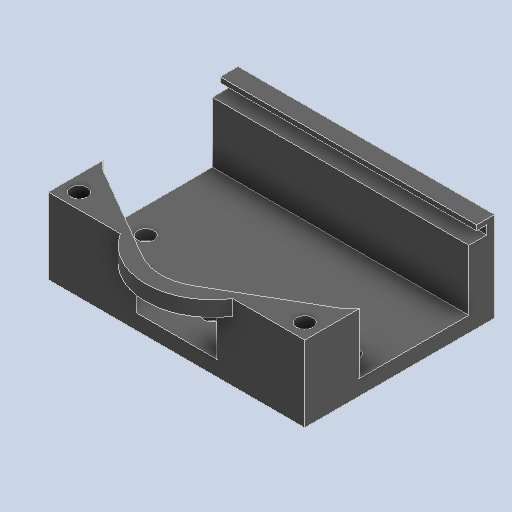
# Autodesk Inventor part: belt_cover_middle
Saved by Autodesk Inventor 2024.1 (Build 281209000, 209)
## iProperties
Created: 2025-02-03
Part Number: belt_cover_middle
Material: 一般
Document SubType Name: モデリング
Designer: hibik
Density: 1 g/cm^3
Appearance: 既定
Sheet Metal Rule: Default_mm
Author: hibik
Autodesk Inventor part; units mm, degrees
ref_plane "YZ Plane" through (0, 0, 0) normal (1, 0, 0) x (0, 1, 0)
ref_plane "XZ Plane" through (0, 0, 0) normal (0, 1, 0) x (-1, 0, 0)
ref_plane "XY Plane" through (0, 0, 0) normal (0, 0, 1) x (1, 0, 0)
sketch "スケッチ1" plane through (0, 0, 0) normal (0, 1, 0) x (-1, 0, 0)
  line L0 (75, 0) -> (105, -51.9615)
  line L1 (-75, 0) -> (-105, -51.9615)
  line L2 (0, -218.2384) -> (0, 36.3731)
  line L3 (147, 0) -> (-147, 0)
  line L4 (105, -51.9615) -> (30, -181.8653)
  line L5 (30, -181.8653) -> (-30, -181.8653)
  line L6 (-30, -181.8653) -> (-105, -51.9615)
  line L7 (75, 0) -> (-75, 0)
  line L8 (34, 0) -> (34, -24.3509)
  line L9 (34, -24.3509) -> (48.7058, -49.822)
  line L10 (48.7058, -49.822) -> (90, -25.9808)
  line L11 (45, 0) -> (45, -18) construction
  line L12 (45, -18) -> (34, -24.3509) construction
  line L13 (84.5, -87.4686) -> (63.4115, -75.2931)
  line L14 (63.4115, -75.2931) -> (48.7058, -49.822)
  line L15 (-34, 0) -> (-34, -24.3509)
  line L16 (-34, -24.3509) -> (-48.7058, -49.822)
  line L17 (-63.4115, -75.2931) -> (-48.7058, -49.822)
  line L18 (-84.5, -87.4686) -> (-63.4115, -75.2931)
  circle A0 centre (30, -32.75) radius 1.6
  circle A1 centre (-30, -32.75) radius 1.6
  line L19 (35.5295, -27) -> (-35.5295, -27)
  point P0 (0, 0)
  point P1 (0, 0)
  point P2 (0, -27)
  dimension "d1" = 150
  dimension "d2" = 60
  dimension "d3" = 60
  dimension "d6" = 60
  dimension "d30" = 60
  dimension "d31" = 18
  dimension "d32" = 30
  dimension "d33" = 41
  dimension "d34" = 3.2
  dimension "d35" = 30
  dimension "d36" = 32.75
  dimension "d37" = 27
  measures "d1" distance of L1.start L0.start
  measures "d2" angle of L3 L0
  measures "d3" angle of L1 L3
  measures "d6" distance of L4.end L5.end
  measures "d30" angle of L11 L12
  measures "d31" distance of L11.start L11.end
  measures "d32" distance of L0.start L11.start
  measures "d33" distance of L0.start L8.start
  measures "d34" diameter of A0
  measures "d35" distance from line of L2 A0.centre
  measures "d36" distance from line of L7 A0.centre
  measures "d37" distance between parallel lines of L7 L19
extrude "プレート1" add sketch "スケッチ1" along normal blind 1.5 contours L14 L13 L4 L5 L2 L19 L9 | L2 L5 L6 L18 L17 L16 L19
sketch "スケッチ4" plane through (0, 1.5, 0) normal (0, 1, 0) x (1, 0, 0)
  circle A0 centre (30, 67.8013) radius 1.6 projected
  circle A1 centre (45, 67.8013) radius 1.6 projected
  line L0 (0, 218.2384) -> (0, -36.3731) projected
  circle A2 centre (-30, 67.8013) radius 1.6
  circle A3 centre (-45, 67.8013) radius 1.6
  line L1 (61.6173, 73.1025) -> (25, 73.1025) projected
  line L2 (25, 73.1025) -> (25, 62.5) projected
  line L3 (-61.6173, 73.1025) -> (-25, 73.1025) projected
  line L4 (-25, 73.1025) -> (-25, 62.5) projected
  line L5 (-25, 62.5) -> (25, 62.5)
  line L6 (-30, 73.1025) -> (30, 73.1025)
  line L7 (30, 73.1025) -> (30, 181.8653)
  line L8 (30, 181.8653) -> (-30, 181.8653)
  line L9 (-30, 181.8653) -> (-30, 73.1025)
  line L10 (-25, 62.5) -> (25, 62.5)
  line L11 (25, 62.5) -> (25, 73.1025)
  line L12 (25, 73.1025) -> (-25, 73.1025)
  line L13 (-25, 73.1025) -> (-25, 62.5)
  line L14 (30, 181.8653) -> (84.5, 87.4686) projected
  line L15 (70, 112.5833) -> (30, 89.4893)
  line L16 (-30, 89.4893) -> (-70, 112.5833)
  line L17 (-84.5, 87.4686) -> (-30, 181.8653) projected
  line L18 (84.5, 87.4686) -> (63.4115, 75.2931) projected
  line L19 (-63.4115, 75.2931) -> (-84.5, 87.4686) projected
  line L20 (-35.5295, 27) -> (-63.4115, 75.2931) projected
  point P0 (0, 0)
  dimension "d40" = 80
  constraints: 22 end point, 6 parallel, 5 point on line, 3 horizontal, 2 centre point, 2 equal radius, 2 perpendicular, 2 symmetric about line, 1 coincident, 1 horizontal alignment
  measures "d40" distance from line of L14.start L15
extrude "切り取り3" cut sketch "スケッチ4" against normal blind 1.5
sketch "スケッチ5" plane through (0, 1.5, 0) normal (0, 1, 0) x (1, 0, 0)
  line L0 (-75, 44) -> (75, 44) projected
  circle A0 centre (-20, 41) radius 3
  circle A1 centre (20, 41) radius 3
  line L1 (-25, 62.5) -> (25, 62.5) projected
  line L2 (0, 62.5) -> (0, 27)
  line L3 (35.5295, 27) -> (-35.5295, 27) projected
  circle A2 centre (-20, 41) radius 1.6
  circle A3 centre (20, 41) radius 1.6
  circle A4 centre (0, 34) radius 1.6
  point P0 (0, 0)
  dimension "d41" = 6
  dimension "d42" = 6
  dimension "d43" = 40
  dimension "d44" = 3.2
  dimension "d45" = 3.2
  dimension "d46" = 3.2
  dimension "d47" = 7
  constraints: 5 centre point, 2 coincident, 2 end point, 2 midpoint, 1 point on line, 1 symmetric about line, 1 tangent
  measures "d41" diameter of A0
  measures "d42" diameter of A1
  measures "d43" distance of A1.centre A0.centre
  measures "d44" diameter of A2
  measures "d45" diameter of A3
  measures "d46" diameter of A4
  measures "d47" vertical distance of A0.centre A4.centre
extrude "切り取り4" cut sketch "スケッチ5" against normal blind 1.5 contours A4 L2 | L2 A4 | A2 | A3
sketch "スケッチ6" plane through (0, 1.5, 0) normal (0, 1, 0) x (1, 0, 0)
  circle A0 centre (-20, 41) radius 1.6 projected
  circle A1 centre (20, 41) radius 1.6 projected
  circle A2 centre (-20, 41) radius 3
  circle A3 centre (20, 41) radius 3
  line L0 (-70.724, 59) -> (85.6586, 59)
  line L1 (85.6586, 59) -> (85.6586, 44)
  line L2 (85.6586, 44) -> (-70.724, 44)
  line L3 (-70.724, 44) -> (-70.724, 59)
  circle A4 centre (0, 34) radius 1.6 projected
  circle A5 centre (0, 34) radius 10
  circle A6 centre (-20, 41) radius 6
  circle A7 centre (20, 41) radius 6
  line L4 (-5.0258, 25.3547) -> (-23.0155, 35.8128)
  line L5 (5.0258, 25.3547) -> (23.0155, 35.8128)
  line L6 (35.5295, 27) -> (-35.5295, 27) projected
  line L7 (-25, 27) -> (-25, 44)
  line L8 (25, 27) -> (25, 44)
  circle A8 centre (-30, 32.75) radius 1.6 projected
  circle A9 centre (30, 32.75) radius 1.6 projected
  line L9 (-25, 73.1025) -> (-25, 62.5) projected
  line L10 (-25, 62.5) -> (-25, 59)
  line L11 (-25, 62.5) -> (25, 62.5) projected
  line L12 (25, 62.5) -> (25, 59)
  point P0 (0, 0)
  point P1 (25, 37.6834)
  point P2 (7.856, 27)
  point P3 (-25, 37.6834)
  point P4 (-7.856, 27)
  dimension "d52" = 12
  dimension "d53" = 12
  dimension "d50" = 6
  dimension "d51" = 15
  dimension "d54" = 5
  dimension "d55" = 5
  constraints: 20 end point, 6 point on line, 5 coincident, 5 perpendicular, 4 tangent, 3 centre point, 2 parallel, 2 point on circle, 1 equal radius, 1 horizontal, 8 other
  measures "d50" diameter of A2
  measures "d51" distance of L0.end L1.end
  measures "d54" distance from line of A8.centre L7
  measures "d55" distance from line of A9.centre L8
extrude "押し出し1" add sketch "スケッチ6" along normal blind 11.8 contours A6 L4 L6 L7 | A7 L8 L6 L5 | L10 L11 L12 L0
sketch "スケッチ7" plane through (0, 1.5, 0) normal (0, 1, 0) x (1, 0, 0)
  line L0 (-176.5784, 180.8905) -> (313.8631, 180.8905)
  line L1 (313.8631, 180.8905) -> (313.8631, -72.7571)
  line L2 (313.8631, -72.7571) -> (-176.5784, -72.7571)
  line L3 (-176.5784, -72.7571) -> (-176.5784, 180.8905)
  point P0 (0, 0)
  constraints: 8 end point, 2 parallel, 1 horizontal, 1 perpendicular
extrude "押し出し2" cut sketch "スケッチ7" against normal through all
sketch "スケッチ8" plane through (25, 13.3, -62.5) normal (0, 0, -1) x (-1, 0, 0)
  line L0 (0, -11.8) -> (50, -11.8) projected
  line L1 (0, -11.8) -> (50, -11.8)
  line L2 (50, -11.8) -> (50, 2.7)
  line L3 (50, 2.7) -> (0, 2.7)
  line L4 (0, 2.7) -> (0, -11.8)
  line L5 (50, -11.8) -> (50, 0) projected
  line L6 (0, 0) -> (50, 0) projected
  point P0 (25, -13.3)
  dimension "d60" = 2.7
  constraints: 8 end point, 2 parallel, 1 collinear, 1 horizontal, 1 perpendicular
  measures "d60" distance between parallel lines of L3 L6
extrude "押し出し3" add sketch "スケッチ8" along normal blind 1.5
sketch "スケッチ9" plane through (25, 13.3, -62.5) normal (0, 0, 1) x (1, 0, 0)
  line L0 (-50, 0) -> (-50, 2.7) projected
  line L1 (-50, 2.7) -> (0, 2.7)
  line L2 (0, 2.7) -> (0, 1.7)
  line L3 (0, 1.7) -> (-50, 1.7)
  line L4 (-50, 1.7) -> (-50, 2.7)
  line L5 (0, 2.7) -> (0, 0) projected
  point P0 (-25, -13.3)
  dimension "d63" = 1
  constraints: 8 end point, 2 parallel, 1 collinear, 1 horizontal, 1 perpendicular
  measures "d63" distance of L1.end L2.end
extrude "押し出し4" add sketch "スケッチ9" along normal blind 2
sketch "スケッチ11" plane through (0, 13.3, 0) normal (0, 1, 0) x (1, 0, 0)
  line L0 (-7.856, 27) -> (-23.0155, 35.8128) projected
  line L1 (23.0155, 35.8128) -> (7.856, 27) projected
  circle A0 centre (0, 34) radius 10
  circle A1 centre (0, 34) radius 13
  line L2 (-7.856, 27) -> (-5.0258, 25.3547)
  line L3 (7.856, 27) -> (5.0258, 25.3547)
  point P0 (0, 0)
  point P1 (-12.2072, 29.5295)
  point P2 (12.2072, 29.5295)
  dimension "d66" = 20
  dimension "d67" = 26
  constraints: 4 end point, 4 tangent, 2 centre point, 2 point on circle, 1 coincident
  measures "d66" diameter of A0
  measures "d67" diameter of A1
extrude "押し出し5" add sketch "スケッチ11" against normal blind 3 contours L2 A0 L3 L1 A1 L0 picked at (-6.6023, 24.0668)
sketch "スケッチ12" plane through (0, 13.3, 0) normal (0, 1, 0) x (1, 0, 0)
  circle A0 centre (-22, 30) radius 1.6
  circle A1 centre (22, 30) radius 1.6
  line L0 (25, 60.5) -> (-25, 60.5) projected
  line L1 (0, 60.5) -> (0, 48.3991)
  line L2 (-25, 27) -> (-10.9545, 27) projected
  line L3 (-25, 37.6834) -> (-25, 27) projected
  point P0 (0, 0)
  dimension "d70" = 3.2
  dimension "d71" = 3
  dimension "d72" = 3
  constraints: 2 centre point, 2 end point, 1 equal radius, 1 midpoint, 1 symmetric about line, 1 vertical
  measures "d70" diameter of A0
  measures "d71" distance from line of L2 A0.centre
  measures "d72" distance from line of L3 A0.centre
extrude "押し出し6" cut sketch "スケッチ12" against normal through all
sketch "スケッチ13" plane through (0, 1.5, 0) normal (0, -1, 0) x (1, 0, 0)
  line L0 (-25, -37.6834) -> (-25, -27) projected
  line L1 (-25, -27) -> (25, -27)
  line L2 (25, -27) -> (25, -64)
  line L3 (25, -64) -> (-25, -64)
  line L4 (-25, -64) -> (-25, -27)
  circle A0 centre (-22, -30) radius 1.6 projected
  circle A1 centre (22, -30) radius 1.6 projected
  point P0 (0, 0)
  constraints: 8 end point, 2 parallel, 1 coincident, 1 horizontal, 1 perpendicular
extrude "押し出し7" add sketch "スケッチ13" along normal blind 2
sketch "スケッチ14" plane through (0, -0.5, 0) normal (0, -1, 0) x (1, 0, 0)
  circle A0 centre (-20, -41) radius 1.6 projected
  circle A1 centre (0, -34) radius 1.6 projected
  circle A2 centre (20, -41) radius 1.6 projected
  line L0 (-30, -73.9008) -> (-76.75, -100.892) projected
  line L1 (-84.5, -87.4686) -> (-76.75, -100.892) projected
  line L2 (-63.4115, -75.2931) -> (-84.5, -87.4686) projected
  line L3 (-35.5295, -27) -> (-63.4115, -75.2931) projected
  line L4 (35.5295, -27) -> (-35.5295, -27) projected
  line L5 (63.4115, -75.2931) -> (35.5295, -27) projected
  line L6 (84.5, -87.4686) -> (63.4115, -75.2931) projected
  line L7 (76.75, -100.892) -> (84.5, -87.4686) projected
  line L8 (76.75, -100.892) -> (30, -73.9008) projected
  line L9 (30, -73.9008) -> (30, -73.1025) projected
  line L10 (30, -73.1025) -> (25, -73.1025) projected
  line L11 (25, -73.1025) -> (25, -62.5) projected
  line L12 (25, -62.5) -> (-25, -62.5) projected
  line L13 (-25, -62.5) -> (-25, -73.1025) projected
  line L14 (-25, -73.1025) -> (-30, -73.1025) projected
  line L15 (-30, -73.1025) -> (-30, -73.9008) projected
  circle A3 centre (-30, -67.8013) radius 1.6 projected
  circle A4 centre (30, -67.8013) radius 1.6 projected
  circle A5 centre (45, -67.8013) radius 1.6 projected
  circle A6 centre (-45, -67.8013) radius 1.6 projected
  circle A7 centre (30, -32.75) radius 1.6 projected
  circle A8 centre (-30, -32.75) radius 1.6 projected
  circle A9 centre (48.4391, -79.9279) radius 1.6 projected
  circle A10 centre (-48.4391, -79.9279) radius 1.6 projected
  circle A11 centre (-73.3666, -93.1522) radius 1.6 projected
  circle A12 centre (73.3666, -93.1522) radius 1.6 projected
  point P0 (0, 0)
extrude "押し出し8" cut sketch "スケッチ14" against normal through all contours A0 | A1 | A2
sketch "スケッチ15" plane through (0, -0.5, 0) normal (0, -1, 0) x (1, 0, 0)
  line L0 (3.2909, -34) -> (1.6454, -36.85)
  line L1 (1.6454, -36.85) -> (-1.6454, -36.85)
  line L2 (-1.6454, -36.85) -> (-3.2909, -34)
  line L3 (-3.2909, -34) -> (-1.6454, -31.15)
  line L4 (-1.6454, -31.15) -> (1.6454, -31.15)
  line L5 (1.6454, -31.15) -> (3.2909, -34)
  line L6 (21.6454, -43.85) -> (18.3546, -43.85)
  line L7 (18.3546, -43.85) -> (16.7091, -41)
  line L8 (16.7091, -41) -> (18.3546, -38.15)
  line L9 (18.3546, -38.15) -> (21.6454, -38.15)
  line L10 (21.6454, -38.15) -> (23.2909, -41)
  line L11 (23.2909, -41) -> (21.6454, -43.85)
  line L12 (-16.7091, -41) -> (-18.3546, -43.85)
  line L13 (-18.3546, -43.85) -> (-21.6454, -43.85)
  line L14 (-21.6454, -43.85) -> (-23.2909, -41)
  line L15 (-23.2909, -41) -> (-21.6454, -38.15)
  line L16 (-21.6454, -38.15) -> (-18.3546, -38.15)
  line L17 (-18.3546, -38.15) -> (-16.7091, -41)
  circle A0 centre (-20, -41) radius 1.6 projected
  circle A1 centre (0, -34) radius 1.6 projected
  circle A2 centre (20, -41) radius 1.6 projected
  circle A3 centre (20, -41) radius 1.6 projected
  circle A4 centre (0, -34) radius 1.6 projected
  circle A5 centre (-20, -41) radius 1.6 projected
  line L18 (25, -64) -> (25, -27) projected
  line L19 (25, -27) -> (-25, -27) projected
  line L20 (-25, -27) -> (-25, -64) projected
  line L21 (-25, -64) -> (25, -64) projected
  circle A6 centre (-22, -30) radius 1.6 projected
  circle A7 centre (22, -30) radius 1.6 projected
  point P0 (0, 0)
  point P1 (0, -34)
  point P2 (20, -41)
  point P3 (-20, -41)
  dimension "d80" = 5.7
  constraints: 36 end point, 3 coincident, 3 horizontal, 2 parallel, 39 other
  measures "d80" distance between parallel lines of L1 L4
extrude "押し出し9" add sketch "スケッチ15" along normal blind 1 contours L21 L20 L19 L18
equation "\"d3\" = d2"
equation "\"d38\" = Thickness"
equation "\"d41\" = d42"
equation "\"d48\" = Thickness"
equation "\"d16\" = Thickness"
equation "\"BendRadius\" = Thickness"
equation "\"BendReliefWidth\" = Thickness"
equation "\"BendReliefDepth\" = 0.5 * Thickness"
equation "\"CornerReliefSize\" = 4 * Thickness"
equation "\"MinimumRemnant\" = 2 * Thickness"
equation "\"TransitionRadius\" = BendRadius"
equation "\"JacobiRadiusSize\" = BendRadius"
equation "\"GapSize\" = Thickness"
equation "\"Thickness\" = 1.5"
